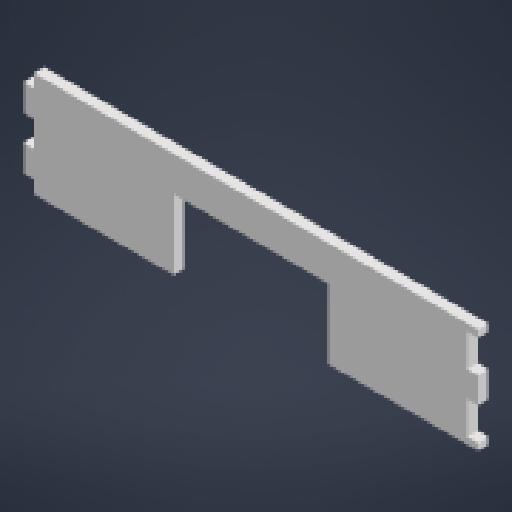
# Autodesk Inventor part: Pieza2
Saved by Autodesk Inventor 2026.1 (Build 301233020, 233B)
## iProperties
Created: 2026-05-06
Part Number: Pieza2
Material: Genérico
Document SubType Name: Modeling
Designer: OlmesTech
Density: 1 g/cm^3
Appearance: Valor por defecto
Author: OlmesTech
Autodesk Inventor part; units mm, degrees
ref_plane "YZ Plane" through (0, 0, 0) normal (1, 0, 0) x (0, 1, 0)
ref_plane "XZ Plane" through (0, 0, 0) normal (0, 1, 0) x (-1, 0, 0)
ref_plane "XY Plane" through (0, 0, 0) normal (0, 0, 1) x (1, 0, 0)
sketch "Boceto1" plane through (0, 0, 0) normal (0, 0, 1) x (1, 0, 0)
  line L0 (45, 15) -> (-82, 15)
  line L1 (45, 15) -> (45, 13.0321)
  line L2 (42, 13.0321) -> (42, 3.7)
  line L3 (42, -13.0321) -> (42, -3.7)
  line L4 (45, 15) -> (45, 13.0321)
  line L5 (45, 3.7) -> (45, 0)
  line L6 (45, 13.0321) -> (45, 15)
  line L7 (45, -15) -> (45, -13.0321)
  line L8 (45, -3.7) -> (45, 3.7)
  line L9 (-82, 15) -> (-82, 11.3)
  line L10 (-85, 11.3) -> (-85, 3.7)
  line L11 (-85, -11.3) -> (-85, -3.7)
  line L12 (-82, 15) -> (-82, 11.3)
  line L13 (-82, 3.7) -> (-82, 0)
  line L14 (-82, 11.3) -> (-82, 15)
  line L15 (-82, -15) -> (-82, -11.3)
  line L16 (-82, -3.7) -> (-82, 3.7)
  line L17 (-85, 11.3) -> (-85, 3.7)
  line L18 (-85, -3.7) -> (-85, -11.3)
  line L19 (45, -15) -> (2, -15)
  line L20 (2, -15) -> (2, 5)
  line L21 (-82, -15) -> (-42, -15)
  line L22 (-42, -15) -> (-42, 5)
  line L23 (-42, 5) -> (2, 5)
  line L24 (42, 13.0321) -> (45, 13.0321)
  line L25 (42, 3.7) -> (45, 3.7)
  line L26 (42, -3.7) -> (45, -3.7)
  line L27 (42, -13.0321) -> (45, -13.0321)
  line L28 (-85, 3.7) -> (-82, 3.7)
  line L29 (-85, -3.7) -> (-82, -3.7)
  line L30 (-85, 11.3) -> (-82, 11.3)
  line L31 (-85, -11.3) -> (-82, -11.3)
  point P0 (-85, 0)
  point P1 (-85, 0)
  dimension "d14" = 3
  dimension "d18" = 3
  dimension "d19" = 3
  dimension "d23" = 130
  dimension "d24" = 43
  dimension "d25" = 20
  dimension "d26" = 40
  dimension "d27" = 43
  constraints: 64 end point, 10 parallel, 7 perpendicular, 2 horizontal, 2 midpoint, 2 vertical
  measures "d14" distance between parallel lines of L10 L13
  measures "d18" distance between parallel lines of L7 L3
  measures "d19" distance between parallel lines of L1 L2
  measures "d23" distance from line of L0.start L10
  measures "d24" distance of L7.start L19.end
  measures "d25" distance of L19.end L20.end
  measures "d26" distance of L15.start L21.end
  measures "d27" distance between parallel lines of L22 L18
extrude "Extrusión1" add sketch "Boceto1" along normal blind 3
